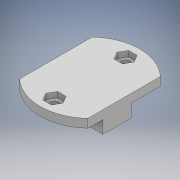
# Autodesk Inventor part: loadCelMountLower
Saved by Autodesk Inventor 2018 (Build 220112000, 112)
## iProperties
Created: 2018-05-09
Part Number: loadCelMountLower
Material: Generic
Document SubType Name: Modeling
Designer: s4321966
Density: 1 g/cm^3
Appearance: Default
Mass: 2.51885 g
Surface Area: 23.0302 cm^2
Volume: 2.51885 cm^3
Author: s4321966
Autodesk Inventor part; units mm, degrees
ref_plane "YZ Plane" through (0, 0, 0) normal (1, 0, 0) x (0, 1, 0)
ref_plane "XZ Plane" through (0, 0, 0) normal (0, 1, 0) x (-1, 0, 0)
ref_plane "XY Plane" through (0, 0, 0) normal (0, 0, 1) x (1, 0, 0)
sketch "Sketch1" plane through (0, 0, 0) normal (0, 0, 1) x (1, 0, 0)
  line L0 (0, 0) -> (4, 0)
  line L1 (4, 0) -> (4, 13)
  line L2 (4, 13) -> (0, 13)
  line L3 (0, 13) -> (0, 0)
  line L4 (4, 13) -> (-4, 13)
  line L5 (-4, 13) -> (-4, -8)
  line L6 (-4, -8) -> (4, -8)
  line L7 (4, -8) -> (4, 13)
  line L8 (-4, 13) -> (4, 13)
  line L9 (4, 13) -> (4, 21)
  line L10 (4, 21) -> (-4, 21)
  line L11 (-4, 21) -> (-4, 13)
  line L12 (4, 21) -> (7, 21)
  line L13 (7, 21) -> (7, 13)
  line L14 (7, 13) -> (4, 13)
  line L15 (4, 13) -> (4, 21)
  line L16 (7, 21) -> (11, 21)
  line L17 (11, 21) -> (11, 13)
  line L18 (11, 13) -> (7, 13)
  line L19 (7, 13) -> (7, 21)
  line L20 (11, 13) -> (4, 13)
  line L21 (4, 13) -> (4, -8)
  line L22 (4, -8) -> (11, -8)
  line L23 (4, -8) -> (11, -8)
  line L24 (11, -8) -> (11, 0)
  line L25 (11, 0) -> (4, 0)
  line L26 (4, 0) -> (4, -8)
  line L27 (11, -8) -> (14, -8)
  line L28 (14, -8) -> (14, 0)
  line L29 (14, 0) -> (11, 0)
  line L30 (11, 0) -> (11, -8)
  line L31 (14, -8) -> (19, -8)
  line L32 (19, -8) -> (19, 13)
  line L33 (19, 13) -> (14, 13)
  line L34 (14, 13) -> (14, -8)
  line L35 (14, 13) -> (22, 13)
  line L36 (14, 18) -> (14, 13)
  line L37 (19, 13) -> (14, 13)
  line L38 (14, 13) -> (14, 21)
  line L39 (14, 21) -> (19, 21)
  line L40 (19, 21) -> (19, 13)
  line L41 (19, -8) -> (-19, -8)
  line L42 (-19, -8) -> (-19, 0)
  line L43 (-19, 0) -> (19, 0)
  line L44 (19, 0) -> (19, -8)
  line L45 (-4, 0) -> (-7, 0)
  line L46 (-7, 0) -> (-7, -8)
  line L47 (-7, -8) -> (-4, -8)
  line L48 (-4, -8) -> (-4, 0)
  line L49 (-7, 0) -> (-11, 0)
  line L50 (-11, 0) -> (-11, -8)
  line L51 (-11, -8) -> (-7, -8)
  line L52 (-7, -8) -> (-7, 0)
  line L53 (-11, -8) -> (-14, -8)
  line L54 (-14, -8) -> (-14, 0)
  line L55 (-14, 0) -> (-11, 0)
  line L56 (-11, 0) -> (-11, -8)
  line L57 (7, 13) -> (11, 13)
  line L58 (11, 13) -> (11, 3)
  line L59 (11, 3) -> (7, 3)
  line L60 (7, 3) -> (7, 13)
  line L61 (-4, 13) -> (-7, 13)
  line L62 (-7, 13) -> (-7, 21)
  line L63 (-7, 21) -> (-4, 21)
  line L64 (-4, 21) -> (-4, 13)
  line L65 (-7, 21) -> (-11, 21)
  line L66 (-11, 21) -> (-11, 13)
  line L67 (-11, 13) -> (-7, 13)
  line L68 (-7, 13) -> (-7, 21)
  line L69 (-7, 13) -> (-11, 13)
  line L70 (-11, 13) -> (-11, 3)
  line L71 (-11, 3) -> (-7, 3)
  line L72 (-7, 3) -> (-7, 13)
  line L73 (-19, -8) -> (-14, -8)
  line L74 (-14, -8) -> (-14, 13)
  line L75 (-14, 13) -> (-19, 13)
  line L76 (-19, 13) -> (-19, -8)
  dimension "d0" = 4
  dimension "d1" = 13
  dimension "d2" = 8
  dimension "d3" = 21
  dimension "d4" = 8
  dimension "d5" = 8
  dimension "d6" = 3
  dimension "d7" = 8
  dimension "d8" = 4
  dimension "d9" = 8
  dimension "d10" = 3
  dimension "d11" = 8
  dimension "d12" = 5
  dimension "d13" = 21
  dimension "d16" = 5
  dimension "d17" = 8
  dimension "d18" = 38
  dimension "d19" = 8
  dimension "d20" = 3
  dimension "d21" = 8
  dimension "d22" = 4
  dimension "d23" = 8
  dimension "d24" = 3
  dimension "d25" = 8
  dimension "d26" = 10
  dimension "d27" = 3
  dimension "d28" = 8
  dimension "d29" = 4
  dimension "d30" = 8
  dimension "d31" = 4
  dimension "d32" = 10
  dimension "d33" = 5
  dimension "d34" = 21
  constraints: 154 end point, 37 parallel, 20 horizontal, 19 perpendicular, 2 point on line
  measures "d0" distance of L2.end L1.end
  measures "d1" distance of L1.end L0.end
  measures "d2" distance of L6.end L5.end
  measures "d3" distance of L5.end L4.end
  measures "d4" distance of L10.end L9.end
  measures "d5" distance of L9.end L8.end
  measures "d6" distance of L13.end L14.end
  measures "d7" distance of L12.end L13.end
  measures "d8" distance of L17.end L18.end
  measures "d9" distance of L16.end L17.end
  measures "d10" distance of L29.end L28.end
  measures "d11" distance of L28.end L27.end
  measures "d12" distance of L33.end L32.end
  measures "d13" distance of L32.end L31.end
  measures "d16" distance of L38.end L39.end
  measures "d17" distance of L37.end L38.end
  measures "d18" distance of L42.end L43.end
  measures "d19" distance of L41.end L42.end
  measures "d20" distance of L47.end L46.end
  measures "d21" distance of L46.end L45.end
  measures "d22" distance of L51.end L50.end
  measures "d23" distance of L50.end L49.end
  measures "d24" distance of L54.end L55.end
  measures "d25" distance of L53.end L54.end
  measures "d26" distance of L57.end L58.end
  measures "d27" distance of L62.end L63.end
  measures "d28" distance of L61.end L62.end
  measures "d29" distance of L67.end L66.end
  measures "d30" distance of L66.end L65.end
  measures "d31" distance of L71.end L70.end
  measures "d32" distance of L70.end L69.end
  measures "d33" distance of L75.end L74.end
  measures "d34" distance of L74.end L73.end
extrude "Extrusion1" add sketch "Sketch1" along normal blind 2.5 contours L3 L2 L1 L0 | L43 L5 L4 L3 | L0 L7 L6 L5 L43 | L25 L24 L22 L7 | L4 L11 L10 L9 L2 | L5 L41 L46 L43 | L9 L12 L13 L14 | L29 L28 L27 L24 | L61 L62 L63 L11 | L46 L41 L50 L43 | L13 L16 L17 L18 | L18 L58 L59 L60 | L43 L32 L31 L28 | L34 L33 L32 L43 | L67 L66 L65 L62 | L72 L71 L70 L67 | L50 L41 L54 L43 | L54 L41 L42 L43 | L43 L76 L75 L74
sketch "Sketch2" plane through (0, 0, 2.5) normal (0, 0, 1) x (1, 0, 0)
  line L0 (-14, 13) -> (-19, 13) projected
  line L1 (-19, 13) -> (-14, 13)
  line L2 (-14, 13) -> (-14, 8)
  line L3 (-14, 8) -> (-19, 8)
  line L4 (-19, 8) -> (-19, 13)
  line L5 (14, 13) -> (19, 13)
  line L6 (19, 13) -> (19, 8)
  line L7 (19, 8) -> (14, 8)
  line L8 (14, 8) -> (14, 13)
  line L9 (-20.5, 6.5) -> (-12.5, 6.5)
  line L10 (-12.5, 6.5) -> (-12.5, 14.5)
  line L11 (-12.5, 14.5) -> (-20.5, 14.5)
  line L12 (-20.5, 14.5) -> (-20.5, 6.5)
  line L13 (12.5, 6.5) -> (20.5, 6.5)
  line L14 (20.5, 6.5) -> (20.5, 14.5)
  line L15 (20.5, 14.5) -> (12.5, 14.5)
  line L16 (12.5, 14.5) -> (12.5, 6.5)
  line L17 (-20.5, 14.5) -> (-19, 14.5)
  line L18 (-19, 14.5) -> (-19, 4.5)
  line L19 (-19, 4.5) -> (-20.5, 4.5)
  line L20 (-20.5, 4.5) -> (-20.5, 14.5)
  line L21 (-14, 0) -> (-14, 13) projected
  line L22 (-12.5, 14.5) -> (-14, 14.5)
  line L23 (-14, 14.5) -> (-14, 4.5)
  line L24 (-14, 4.5) -> (-12.5, 4.5)
  line L25 (-12.5, 4.5) -> (-12.5, 14.5)
  line L26 (-19, 14.5) -> (-14, 14.5)
  line L27 (-14, 14.5) -> (-14, 13)
  line L28 (-14, 13) -> (-19, 13)
  line L29 (-19, 13) -> (-19, 14.5)
  line L30 (12.5, 14.5) -> (20.5, 14.5)
  line L31 (20.5, 14.5) -> (20.5, 13)
  line L32 (20.5, 13) -> (12.5, 13)
  line L33 (12.5, 13) -> (12.5, 14.5)
  line L34 (14, 13) -> (14, 0) projected
  line L35 (12.5, 14.5) -> (14, 14.5)
  line L36 (14, 14.5) -> (14, 4.5)
  line L37 (14, 4.5) -> (12.5, 4.5)
  line L38 (12.5, 4.5) -> (12.5, 14.5)
  line L39 (19, -8) -> (19, 13) projected
  line L40 (20.5, 14.5) -> (19, 14.5)
  line L41 (19, 14.5) -> (19, 4.5)
  line L42 (19, 4.5) -> (20.5, 4.5)
  line L43 (20.5, 4.5) -> (20.5, 14.5)
  point P0 (0, 0)
  dimension "d37" = 5
  dimension "d38" = 5
  dimension "d39" = 5
  dimension "d40" = 5
  dimension "d41" = 1.5
  dimension "d42" = 1.5
  dimension "d43" = 1.5
  dimension "d44" = 10
  dimension "d45" = 10
  dimension "d46" = 10
  constraints: 80 end point, 20 parallel, 10 perpendicular, 8 horizontal, 6 point on line, 6 other
  measures "d37" distance of L2.end L3.end
  measures "d38" distance of L1.end L2.end
  measures "d39" distance of L6.end L7.end
  measures "d40" distance of L5.end L6.end
  measures "d41" distance between parallel lines of L3 L9
  measures "d42" distance between parallel lines of L7 L13
  measures "d43" distance of L18.end L19.end
  measures "d44" distance of L17.end L18.end
  measures "d45" distance of L35.end L36.end
  measures "d46" distance of L41.end L40.end
extrude "Extrusion2" add sketch "Sketch2" along normal blind 3 contours L23 L11 L10 L9 L21 L2 | L0 L18 L11 L23 | L4 L18 L9 L12 L11 | L9 L25 L24 L21 | L18 L19 L20 L9 | L36 L15 L41 L5 | L8 L34 L13 L16 L32 | L32 L16 L15 L36 | L32 L14 L13 L39 L6 | L41 L15 L14 L32 | L34 L37 L38 L13 | L13 L43 L42 L39
sketch "Sketch4" plane through (0, 0, 5.5) normal (0, 0, 1) x (1, 0, 0)
  line L0 (-12.5, 14.5) -> (-20.5, 14.5) projected
  line L1 (-12.5, 4.5) -> (-12.5, 14.5) projected
  line L2 (-20.5, 14.5) -> (-12.5, 14.5)
  line L3 (-12.5, 14.5) -> (-12.5, 4.5)
  line L4 (-12.5, 4.5) -> (-20.5, 4.5)
  line L5 (-20.5, 4.5) -> (-20.5, 14.5)
  line L6 (12.5, 14.5) -> (12.5, 4.5) projected
  line L7 (20.5, 4.5) -> (20.5, 14.5) projected
  line L8 (12.5, 14.5) -> (20.5, 14.5)
  line L9 (20.5, 14.5) -> (20.5, 4.5)
  line L10 (20.5, 4.5) -> (12.5, 4.5)
  line L11 (12.5, 4.5) -> (12.5, 14.5)
  point P0 (0, 0)
  constraints: 16 end point, 4 parallel, 2 horizontal, 2 perpendicular
extrude "Extrusion3" add sketch "Sketch4" along normal blind 1.5
sketch "Sketch5" plane through (0, 0, 7) normal (0, 0, 1) x (1, 0, 0)
  line L0 (-12.5, 14.5) -> (-20.5, 14.5) projected
  line L1 (20.5, 4.5) -> (20.5, 14.5) projected
  line L2 (-20.5, 14.5) -> (20.5, 14.5)
  line L3 (20.5, 14.5) -> (20.5, 4.5)
  line L4 (20.5, 4.5) -> (-20.5, 4.5)
  line L5 (-20.5, 4.5) -> (-20.5, 14.5)
  line L6 (-20.5, 14.5) -> (-20.5, 4.5) projected
  line L7 (-20.5, 9.5) -> (20.5, 9.5)
  line L8 (0, 9.5) -> (0, 14.5)
  circle A0 centre (0, 9.5) radius 17.5
  point P0 (0, 0)
  constraints: 12 end point, 4 midpoint, 2 parallel, 1 centre point, 1 coincident, 1 horizontal, 1 perpendicular
extrude "Extrusion4" add sketch "Sketch5" along normal blind 1.5
sketch "Sketch6" plane through (0, 0, 8.5) normal (0, 0, 1) x (1, 0, 0)
  arc A0 (16.7705, 14.5) -> (-16.7705, 14.5) centre (0, 9.5) ccw projected
  circle A1 centre (0, 9.5) radius 17.5
  circle A2 centre (0, 9.5) radius 7.5
  circle A3 centre (0, 9.5) radius 12.5
  line L0 (12.5, 14.5) -> (12.5, 4.5) projected
  circle A4 centre (0, 9.5) radius 10
  circle A5 centre (0, -0.5) radius 1.651
  circle A6 centre (0, 2) radius 1.651
  circle A7 centre (7.5, 9.5) radius 1.651
  circle A8 centre (-7.5, 9.5) radius 1.651
  circle A9 centre (0, 17) radius 1.651
  circle A10 centre (0, 22) radius 1.651
  circle A11 centre (0, -3) radius 1.651
  point P0 (0, 0)
  dimension "d54" = 20
  dimension "d53" = 15
  dimension "d55" = 3.302
  dimension "d56" = 3.302
  dimension "d57" = 3.302
  dimension "d58" = 3.302
  dimension "d59" = 3.302
  dimension "d62" = 3.302
  dimension "d63" = 3.302
  constraints: 9 centre point, 6 point on circle, 4 coincident, 1 tangent, 1 vertical alignment, 5 other
  measures "d53" diameter of A2
  measures "d55" diameter of A5
  measures "d56" diameter of A6
  measures "d57" diameter of A7
  measures "d58" diameter of A8
  measures "d59" diameter of A9
  measures "d62" diameter of A10
  measures "d63" diameter of A11
extrude "Extrusion5" cut sketch "Sketch6" against normal blind 2.5 contours A2 A7 | A2 A7 | A8 A2 | A2 A8 | A11 A5 | A5 A11 A3 | A3 A11 | A10 A3 | A3 A10
sketch "Sketch7" plane through (0, 0, 2.5) normal (0, 0, -1) x (-1, 0, 0)
  line L0 (-36.0395, -19.2499) -> (42.4279, -19.2499)
  line L1 (42.4279, -19.2499) -> (42.4279, 35.743)
  line L2 (42.4279, 35.743) -> (-36.0395, 35.743)
  line L3 (-36.0395, 35.743) -> (-36.0395, -19.2499)
  point P0 (0, 0)
  constraints: 8 end point, 2 parallel, 1 horizontal, 1 perpendicular
extrude "Extrusion6" cut sketch "Sketch7" along normal blind 2.5
sketch "Sketch8" plane through (0, 0, 2.5) normal (0, 0, -1) x (-1, 0, 0)
  line L0 (-12.5, 14.5) -> (-12.5, 4.5) projected
  line L1 (-12.5, 14.5) -> (-13, 14.5)
  line L2 (-13, 14.5) -> (-13, 4.5)
  line L3 (-13, 4.5) -> (-12.5, 4.5)
  line L4 (-12.5, 4.5) -> (-12.5, 14.5)
  line L5 (12.5, 4.5) -> (12.5, 14.5) projected
  line L6 (12.5, 14.5) -> (13, 14.5)
  line L7 (13, 14.5) -> (13, 4.5)
  line L8 (13, 4.5) -> (12.5, 4.5)
  line L9 (12.5, 4.5) -> (12.5, 14.5)
  point P0 (0, 0)
  dimension "d66" = 0.5
  dimension "d67" = 10
  dimension "d68" = 0.5
  dimension "d69" = 10
  constraints: 16 end point, 4 parallel, 2 horizontal, 2 perpendicular
  measures "d66" distance of L3.end L2.end
  measures "d67" distance of L2.end L1.end
  measures "d68" distance of L7.end L8.end
  measures "d69" distance of L6.end L7.end
extrude "Extrusion7" cut sketch "Sketch8" against normal blind 4.5
sketch "Sketch10" plane through (0, 0, 2.5) normal (0, 0, -1) x (-1, 0, 0)
  line L0 (19, 13) -> (19, 4.5) projected
  line L1 (19, 13) -> (14, 13)
  line L2 (14, 13) -> (14, -8)
  line L3 (14, -8) -> (19, -8)
  line L4 (19, -8) -> (19, 13)
  line L5 (14, -8) -> (11, -8)
  line L6 (11, -8) -> (11, 0)
  line L7 (11, 0) -> (14, 0)
  line L8 (14, 0) -> (14, -8)
  line L9 (11, -8) -> (7, -8)
  line L10 (7, -8) -> (7, 0)
  line L11 (7, 0) -> (11, 0)
  line L12 (11, 0) -> (11, -8)
  line L13 (7, -8) -> (4, -8)
  line L14 (4, -8) -> (4, 0)
  line L15 (4, 0) -> (7, 0)
  line L16 (7, 0) -> (7, -8)
  line L17 (4, -8) -> (0, -8)
  line L18 (0, -8) -> (0, 0)
  line L19 (0, 0) -> (4, 0)
  line L20 (4, 0) -> (4, -8)
  line L21 (0, 0) -> (-4, 0)
  line L22 (-4, 0) -> (-4, -8)
  line L23 (-4, -8) -> (0, -8)
  line L24 (0, -8) -> (0, 0)
  line L25 (-4, -8) -> (-7, -8)
  line L26 (-7, -8) -> (-7, 0)
  line L27 (-7, 0) -> (-4, 0)
  line L28 (-4, 0) -> (-4, -8)
  line L29 (-7, -8) -> (-11, -8)
  line L30 (-11, -8) -> (-11, 0)
  line L31 (-11, 0) -> (-7, 0)
  line L32 (-7, 0) -> (-7, -8)
  line L33 (-11, -8) -> (-14, -8)
  line L34 (-14, -8) -> (-14, 0)
  line L35 (-14, 0) -> (-11, 0)
  line L36 (-11, 0) -> (-11, -8)
  line L37 (-14, -8) -> (-19, -8)
  line L38 (-19, -8) -> (-19, 13)
  line L39 (-19, 13) -> (-14, 13)
  line L40 (-14, 13) -> (-14, -8)
  line L41 (4, -8) -> (-4, -8)
  line L42 (-4, -8) -> (-4, 21)
  line L43 (-4, 21) -> (4, 21)
  line L44 (4, 21) -> (4, -8)
  line L45 (4, 21) -> (7, 21)
  line L46 (7, 21) -> (7, 13)
  line L47 (7, 13) -> (4, 13)
  line L48 (4, 13) -> (4, 21)
  line L49 (-4, 21) -> (-7, 21)
  line L50 (-7, 21) -> (-7, 13)
  line L51 (-7, 13) -> (-4, 13)
  line L52 (-4, 13) -> (-4, 21)
  line L53 (4, 0) -> (14, 0)
  line L54 (14, 0) -> (14, 3)
  line L55 (14, 3) -> (4, 3)
  line L56 (4, 3) -> (4, 0)
  line L57 (7, 13) -> (4, 13)
  line L58 (4, 13) -> (4, 3)
  line L59 (4, 3) -> (7, 3)
  line L60 (7, 3) -> (7, 13)
  line L61 (7, 3) -> (12, 3)
  line L62 (12, 3) -> (12, 13)
  line L63 (12, 13) -> (7, 13)
  line L64 (7, 13) -> (7, 3)
  line L65 (12, 13) -> (7, 13)
  line L66 (7, 13) -> (7, 21)
  line L67 (7, 21) -> (12, 21)
  line L68 (12, 21) -> (12, 13)
  line L69 (7, 3) -> (11, 3)
  line L70 (11, 3) -> (11, 21)
  line L71 (11, 21) -> (7, 21)
  line L72 (7, 21) -> (7, 3)
  line L73 (-7, 21) -> (-11, 21)
  line L74 (-11, 21) -> (-11, 8)
  line L75 (-11, 8) -> (-7, 8)
  line L76 (-7, 8) -> (-7, 21)
  line L77 (-11, 8) -> (-7, 8)
  line L78 (-7, 8) -> (-7, 3)
  line L79 (-7, 3) -> (-11, 3)
  line L80 (-11, 3) -> (-11, 8)
  dimension "d72" = 5
  dimension "d73" = 21
  dimension "d74" = 3
  dimension "d75" = 8
  dimension "d76" = 4
  dimension "d77" = 8
  dimension "d78" = 3
  dimension "d79" = 8
  dimension "d80" = 4
  dimension "d81" = 3
  dimension "d82" = 8
  dimension "d83" = 4
  dimension "d84" = 8
  dimension "d85" = 3
  dimension "d86" = 8
  dimension "d87" = 5
  dimension "d88" = 21
  dimension "d89" = 8
  dimension "d90" = 29
  dimension "d91" = 3
  dimension "d92" = 8
  dimension "d93" = 3
  dimension "d94" = 5
  dimension "d95" = 10
  dimension "d96" = 4
  dimension "d97" = 4
  dimension "d98" = 13
  dimension "d99" = 5
  constraints: 160 end point, 40 parallel, 20 horizontal, 20 perpendicular, 5 point on line
  measures "d72" distance of L3.end L2.end
  measures "d73" distance of L2.end L1.end
  measures "d74" distance of L6.end L7.end
  measures "d75" distance of L5.end L6.end
  measures "d76" distance of L10.end L11.end
  measures "d77" distance of L9.end L10.end
  measures "d78" distance of L14.end L15.end
  measures "d79" distance of L13.end L14.end
  measures "d80" distance of L23.end L22.end
  measures "d81" distance of L26.end L27.end
  measures "d82" distance of L25.end L26.end
  measures "d83" distance of L30.end L31.end
  measures "d84" distance of L29.end L30.end
  measures "d85" distance of L34.end L35.end
  measures "d86" distance of L33.end L34.end
  measures "d87" distance of L38.end L39.end
  measures "d88" distance of L37.end L38.end
  measures "d89" distance of L42.end L43.end
  measures "d90" distance of L41.end L42.end
  measures "d91" distance of L46.end L47.end
  measures "d92" distance of L45.end L46.end
  measures "d93" distance of L54.end L53.end
  measures "d94" distance of L63.end L62.end
  measures "d95" distance of L62.end L61.end
  measures "d96" distance of L71.end L70.end
  measures "d97" distance of L75.end L74.end
  measures "d98" distance of L74.end L73.end
  measures "d99" distance of L77.end L78.end
extrude "Extrusion8" add sketch "Sketch10" along normal blind 2.5 contours L55 L70 L63 L62 | L55 L60 L63 L70 | L78 L79 L80 L75
sketch "Sketch12" plane through (0, 0, 2.5) normal (0, 0, -1) x (-1, 0, 0)
  line L0 (-20.5, 14.5) -> (-16.7705, 14.5) projected
  line L1 (-13, 4.5) -> (-14, 4.5) projected
  line L2 (-13, 4.5) -> (-20.5, 4.5)
  line L3 (-20.5, 4.5) -> (-20.5, 14.5)
  line L4 (-20.5, 14.5) -> (-20.5, 4.5)
  line L5 (-20.5, 4.5) -> (-20.5, 14.5) projected
  line L6 (-20.5, 14.5) -> (-20.5, 4.5)
  line L7 (-11, 3) -> (-7, 3) projected
  line L8 (-11, 3) -> (-7, 3)
  line L9 (7, 3) -> (12, 3) projected
  line L10 (7, 3) -> (11, 3)
  line L11 (-6, 2) -> (-12, 2)
  line L12 (6, 2) -> (12, 2)
  line L13 (-11, 3) -> (-12, 3)
  line L14 (-12, 2) -> (-11, 2)
  line L15 (-11, 2) -> (-11, 12)
  line L16 (-11, 12) -> (-12, 12)
  line L17 (-12, 12) -> (-12, 2)
  line L18 (-6, 2) -> (-7, 2)
  line L19 (-7, 2) -> (-7, 12)
  line L20 (-7, 12) -> (-6, 12)
  line L21 (-6, 12) -> (-6, 2)
  line L22 (-11, 3) -> (-7, 3)
  line L23 (-7, 3) -> (-7, 2)
  line L24 (-7, 2) -> (-11, 2)
  line L25 (-11, 2) -> (-11, 3)
  line L26 (6, 2) -> (7, 2)
  line L27 (7, 2) -> (7, 12)
  line L28 (7, 12) -> (6, 12)
  line L29 (6, 12) -> (6, 2)
  line L30 (12, 2) -> (11, 2)
  line L31 (11, 2) -> (11, 12)
  line L32 (11, 12) -> (12, 12)
  line L33 (12, 12) -> (12, 2)
  line L34 (11, 2) -> (7, 2)
  line L35 (7, 2) -> (7, 3)
  line L36 (7, 3) -> (11, 3)
  line L37 (11, 3) -> (11, 2)
  point P0 (0, 0)
  dimension "d102" = 10
  dimension "d108" = 10
  dimension "d109" = 10
  dimension "d110" = 10
  dimension "d111" = 10
  constraints: 66 end point, 13 equal length, 9 horizontal, 7 perpendicular
  measures "d102" distance of L0.start L2.end
  measures "d108" distance of L15.end L14.end
  measures "d109" distance of L18.end L19.end
  measures "d110" distance of L27.end L26.end
  measures "d111" distance of L30.end L31.end
extrude "Extrusion9" add sketch "Sketch12" against normal blind 4.5
sketch "Sketch13" plane through (0, 0, 2.5) normal (0, 0, -1) x (-1, 0, 0)
  line L0 (-38.1757, -13.5793) -> (29.0802, -13.5793)
  line L1 (29.0802, -13.5793) -> (29.0802, 23.5075)
  line L2 (29.0802, 23.5075) -> (-38.1757, 23.5075)
  line L3 (-38.1757, 23.5075) -> (-38.1757, -13.5793)
  point P0 (0, 0)
  constraints: 8 end point, 2 parallel, 1 horizontal, 1 perpendicular
extrude "Extrusion10" cut sketch "Sketch13" along normal blind 4.5
sketch "Sketch15" plane through (0, 0, 7) normal (0, 0, -1) x (-1, 0, 0)
  line L0 (-11, 12) -> (-11, 3) projected
  line L1 (-7, 12) -> (-6, 12) projected
  line L2 (-11, 3) -> (-7, 3)
  line L3 (-7, 3) -> (-7, 12)
  line L4 (-7, 12) -> (-11, 12)
  line L5 (-11, 12) -> (-11, 3)
  line L6 (7, 7.9265) -> (7, 3) projected
  line L7 (11, 12) -> (11, 3) projected
  line L8 (7, 3) -> (11, 3)
  line L9 (11, 3) -> (11, 12)
  line L10 (11, 12) -> (7, 12)
  line L11 (7, 12) -> (7, 3)
  point P0 (0, 0)
  constraints: 16 end point, 4 parallel, 2 horizontal, 2 perpendicular
extrude "Extrusion11" add sketch "Sketch15" along normal blind 1.5
sketch "Sketch16" plane through (0, 0, 7) normal (0, 0, -1) x (-1, 0, 0)
  line L0 (-12.4141, 17.8254) -> (-32.5951, 17.8254)
  line L1 (-32.5951, 17.8254) -> (-32.5951, -1.1459)
  line L2 (-32.5951, -1.1459) -> (-12.4141, -1.1459)
  line L3 (-12.4141, -1.1459) -> (-12.4141, 17.8254)
  line L4 (12.4778, 16.3612) -> (30.5579, 16.3612)
  line L5 (30.5579, 16.3612) -> (30.5579, -3.4378)
  line L6 (30.5579, -3.4378) -> (12.4778, -3.4378)
  line L7 (12.4778, -3.4378) -> (12.4778, 16.3612)
  point P0 (0, 0)
  constraints: 16 end point, 4 parallel, 2 horizontal, 2 perpendicular
extrude "Extrusion12" cut sketch "Sketch16" along normal blind 10
sketch "Sketch17" plane through (0, 0, 7) normal (0, 0, -1) x (-1, 0, 0)
  arc A0 (16.7705, 14.5) -> (-16.7705, 14.5) centre (0, 9.5) ccw projected
  circle A1 centre (0, 9.5) radius 17.5
  circle A2 centre (0, 9.5) radius 24.0818
  point P0 (0, 0)
  constraints: 2 coincident, 1 centre point, 3 other
extrude "Extrusion13" cut sketch "Sketch17" against normal blind 10
sketch "Sketch18" plane through (0, 9.5, 8.5) normal (0, 0, 1) x (1, 0, 0)
  line L0 (12.6688, -5.8076) -> (-12.9871, -5.8076)
  line L1 (-12.9871, -5.8076) -> (-12.9871, 4.3147)
  line L2 (-12.9871, 4.3147) -> (12.6688, 4.3147)
  line L3 (12.6688, 4.3147) -> (12.6688, -5.8076)
  point P0 (0, -9.5)
  constraints: 8 end point, 2 parallel, 1 horizontal, 1 perpendicular
extrude "Extrusion14" add sketch "Sketch18" against normal blind 1.5
sketch "Sketch19" plane through (0, 9.5, 7) normal (0, 0, -1) x (-1, 0, 0)
  line L0 (-12, -7.5) -> (-12, 2.5) projected
  line L1 (-12, -2.5) -> (-30.6852, -2.5)
  line L2 (-30.6852, -2.5) -> (-30.6852, 13.7367)
  line L3 (-30.6852, 13.7367) -> (-12, 13.7367)
  line L4 (-12, 13.7367) -> (-12, -2.5)
  line L5 (12, 2.5) -> (12, -7.5) projected
  line L6 (12, -2.5) -> (23.555, -2.5)
  line L7 (23.555, -2.5) -> (23.555, -20.9592)
  line L8 (23.555, -20.9592) -> (12, -20.9592)
  line L9 (12, -20.9592) -> (12, -2.5)
  line L10 (-12, 13.7367) -> (-34.1229, 13.7367)
  line L11 (-34.1229, 13.7367) -> (-34.1229, -29.7446)
  line L12 (-34.1229, -29.7446) -> (-12, -29.7446)
  line L13 (-12, -29.7446) -> (-12, 13.7367)
  line L14 (12, -17.0758) -> (29.03, -17.0758)
  line L15 (29.03, -17.0758) -> (29.03, 15.9012)
  line L16 (29.03, 15.9012) -> (12, 15.9012)
  line L17 (12, 15.9012) -> (12, -17.0758)
  point P0 (0, -9.5)
  constraints: 32 end point, 8 parallel, 4 horizontal, 4 perpendicular, 2 midpoint, 1 point on line
extrude "Extrusion15" cut sketch "Sketch19" against normal blind 1.5
sketch "Sketch23" plane through (0, 0, 8.5) normal (0, 0, 1) x (1, 0, 0)
  circle A0 centre (0, 22) radius 1.651 projected
  circle A1 centre (0, 22) radius 3
  circle A2 centre (0, -3) radius 1.651 projected
  circle A3 centre (0, -3) radius 3
  line L0 (3, 22) -> (1.5, 19.4019)
  line L1 (1.5, 19.4019) -> (-1.5, 19.4019)
  line L2 (-1.5, 19.4019) -> (-3, 22)
  line L3 (-3, 22) -> (-1.5, 24.5981)
  line L4 (-1.5, 24.5981) -> (1.5, 24.5981)
  line L5 (1.5, 24.5981) -> (3, 22)
  line L6 (3, -3) -> (1.5, -5.5981)
  line L7 (1.5, -5.5981) -> (-1.5, -5.5981)
  line L8 (-1.5, -5.5981) -> (-3, -3)
  line L9 (-3, -3) -> (-1.5, -0.4019)
  line L10 (-1.5, -0.4019) -> (1.5, -0.4019)
  line L11 (1.5, -0.4019) -> (3, -3)
  line L12 (12, -3.2377) -> (12, 22.2377) projected
  line L13 (-12, 22.2377) -> (-12, -3.2377) projected
  arc A4 (12, 22.2377) -> (-12, 22.2377) centre (0, 9.5) ccw
  arc A5 (-12, -3.2377) -> (12, -3.2377) centre (0, 9.5) ccw
  line L14 (12, 22.2377) -> (12, -3.2377)
  arc A6 (12, 22.2377) -> (-12, 22.2377) centre (0, 9.5) ccw projected
  line L15 (-12, 22.2377) -> (-12, -3.2377)
  point P0 (0, 0)
  dimension "d130" = 6
  dimension "d131" = 6
  constraints: 28 end point, 4 coincident, 4 point on circle, 2 centre point, 2 horizontal alignment, 1 collinear, 30 other
extrude "Extrusion17" add sketch "Sketch23" along normal blind 1.5 contours L5 A1 | A1 L0 | L4 A1 | A1 L1 | L3 A1 | A1 L2 | L11 A3 | A3 L6 | L10 A3 | A3 L7 | L9 A3 | A3 L8 | A5 L13 A4 L12
sketch "Sketch24" plane through (0, 0, 8.5) normal (0, 0, 1) x (1, 0, 0)
  circle A0 centre (0, 22) radius 1.651 projected
  circle A1 centre (0, 22) radius 1.651
  circle A2 centre (0, -3) radius 1.651 projected
  circle A3 centre (0, -3) radius 1.651
  line L0 (1.5, 19.4019) -> (3, 22) projected
  line L1 (3, 22) -> (1.5, 19.4019)
  line L2 (1.5, 19.4019) -> (-1.5, 19.4019)
  line L3 (-1.5, 19.4019) -> (-3, 22)
  line L4 (-3, 22) -> (-1.5, 24.5981)
  line L5 (-1.5, 24.5981) -> (1.5, 24.5981)
  line L6 (1.5, 24.5981) -> (3, 22)
  line L7 (3, -3) -> (1.5, -5.5981)
  line L8 (1.5, -5.5981) -> (-1.5, -5.5981)
  line L9 (-1.5, -5.5981) -> (-3, -3)
  line L10 (-3, -3) -> (-1.5, -0.4019)
  line L11 (-1.5, -0.4019) -> (1.5, -0.4019)
  line L12 (1.5, -0.4019) -> (3, -3)
  point P0 (0, 0)
  constraints: 24 end point, 4 coincident, 2 centre point, 26 other
extrude "Extrusion18" cut sketch "Sketch24" against normal blind 0.5
body "Solid1"
